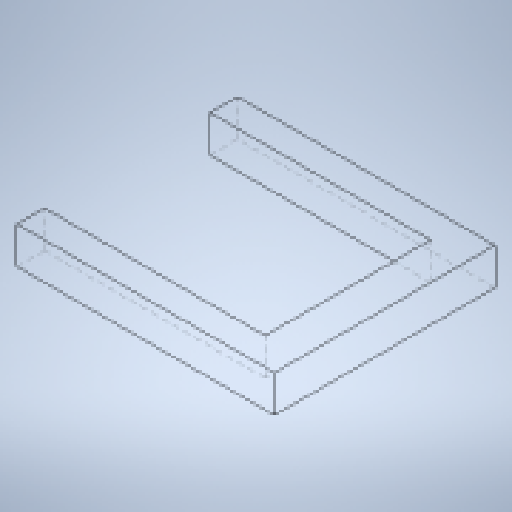
# Autodesk Inventor part: Rack
Saved by Autodesk Inventor 2023.2 (Build 272271000, 271)
## iProperties
Created: 2024-01-11
Part Number: Rack
Material: Aluminum 6061
Document SubType Name: Modeling
Designer: Nathan Cai
Mass: 25.5792 g
Surface Area: 51.4053 cm^2
Volume: 9.47377 cm^3
Density: 2.7 g/cm^3
Appearance: Aluminum - Flat
Author: Nathan Cai
Autodesk Inventor part; units mm, degrees
ref_plane "YZ Plane" through (0, 0, 0) normal (1, 0, 0) x (0, 1, 0)
ref_plane "XZ Plane" through (0, 0, 0) normal (0, 1, 0) x (-1, 0, 0)
ref_plane "XY Plane" through (0, 0, 0) normal (0, 0, 1) x (1, 0, 0)
sketch "Sketch1" plane through (0, 0, 0) normal (0, 1, 0) x (-1, 0, 0)
  line L0 (25.4, 26.9875) -> (-25.4, 26.9875)
  line L1 (-25.4, 26.9875) -> (-25.4, -26.9875)
  line L2 (-25.4, -26.9875) -> (25.4, -26.9875)
  line L3 (25.4, -26.9875) -> (25.4, 26.9875)
  line L4 (25.4, 26.9875) -> (-25.4, -26.9875) construction
  line L5 (-25.4, 26.9875) -> (25.4, -26.9875) construction
  line L6 (0, 0) -> (-25.4, 0) construction
  line L7 (25.4, 33.3375) -> (-38.1, 33.3375)
  line L8 (-38.1, 33.3375) -> (-38.1, -33.3375)
  line L9 (-38.1, -33.3375) -> (25.4, -33.3375)
  line L10 (25.4, -33.3375) -> (25.4, 33.3375)
  line L11 (25.4, 33.3375) -> (-38.1, -33.3375) construction
  line L12 (-38.1, 33.3375) -> (25.4, -33.3375) construction
  point P0 (-6.35, 0)
  point P1 (25.4, 26.9875)
  dimension "d0" = 50.8
  dimension "d1" = 53.975
  dimension "d2" = 6.35
  dimension "d3" = 12.7
  constraints: 26 end point, 5 midpoint, 4 parallel, 2 horizontal, 2 perpendicular, 2 point on line
  measures "d0" distance of L2.end L1.end
  measures "d1" distance of L1.end L0.end
  measures "d2" distance between parallel lines of L2 L9
  measures "d3" distance between parallel lines of L1 L8
extrude "Extrusion1" add sketch "Sketch1" along normal blind 6.35 contours L0 L1 L2 L10 L9 L8 L7
chamfer "Chamfer1" distance 9.525 angle 45 4 edges at (25.4, 3.175, 26.9875) (38.1, 3.175, 33.3375) (25.4, 3.175, -26.9875) (38.1, 3.175, -33.3375)
body "Solid1"
